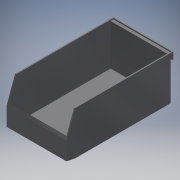
# Autodesk Inventor part: 22-124
Saved by Autodesk Inventor 2018 (Build 220105000, 105)
## iProperties
Created: 2004-11-24
Part Number: 22-124
Document SubType Name: Modeling
Designer: Autodesk, Inc.
Manufacturer: Standard
Standards Organization: Custom
Description: Parts Bin, Conductive, Small
Vendor: PARKER IPS
Catalog Web Link: http://www.parker.com/ead/cm1.asp?cmid=809
Mass: 114.974 g
Surface Area: 1166.8 cm^2
Volume: 114.974 cm^3
Density: 1 g/cm^3
Material: Generic
Appearance: Smooth - Medium Gray
CAGE: 1LJX3
Dept. ID: Product Design
Description #2: ---
Finish #1: ---
Finish #2: ---
Material ID: ---
Project Number: ---
Author: Autodesk, Inc.
Autodesk Inventor part; units mm, degrees
ref_plane "YZ Plane" through (0, 0, 0) normal (1, 0, 0) x (0, 1, 0)
ref_plane "XZ Plane" through (0, 0, 0) normal (0, 1, 0) x (-1, 0, 0)
ref_plane "XY Plane" through (0, 0, 0) normal (0, 0, 1) x (1, 0, 0)
sketch "Sketch2" plane through (0, 0, 0) normal (1, 0, 0) x (0, 1, 0)
  line L0 (-33.0843, 98.5) -> (-2.0843, 98.5)
  line L1 (-2.0843, 98.5) -> (40, 83.5)
  line L2 (40, 83.5) -> (40, -88.5)
  line L3 (40, -88.5) -> (28, -88.5)
  line L4 (28, -88.5) -> (28, -86.5)
  line L5 (28, -86.5) -> (36, -86.5)
  line L6 (36, -86.5) -> (36, -83.5)
  line L7 (36, -83.5) -> (-36, -83.5)
  line L8 (-36, -83.5) -> (-36, 83.5)
  line L9 (-36, 83.5) -> (-33.0843, 98.5)
  point P0 (0, 0)
  point P1 (0, -83.5)
  point P2 (-36, 0)
  dimension "d0" = 15
  dimension "d1" = 11
  dimension "d2" = 31
  dimension "d4" = 2
  dimension "d5" = 3
  dimension "d6" = 4
  dimension "d7" = 12
  dimension "Dim_D" = 187
  dimension "Dim_H" = 76
  dimension "d11" = 19.617
  dimension "d12" = 15
  constraints: 20 end point, 5 parallel, 2 midpoint, 2 perpendicular, 1 horizontal, 1 horizontal alignment, 1 vertical alignment
  measures "d0" vertical distance of L8.end L0.start
  measures "d1" angle of L8 L9
  measures "d2" distance of L0.start L0.end
  measures "d4" distance of L3.end L4.end
  measures "d5" distance between parallel lines of L7 L5
  measures "d6" distance between parallel lines of L2 L6
  measures "d7" distance of L2.end L3.end
  measures "Dim_D" distance between parallel lines of L3 L0
  measures "Dim_H" distance between parallel lines of L8 L2
  measures "d11" angle of L1 L0
  measures "d12" vertical distance of L0.end L1.end
extrude "Extrusion1" add sketch "Sketch2" along normal mid plane 105
shell "Shell1" thickness 2 removed faces 2 at (-17.5, 25.9719, 88.5) at (-17.5, 40, -31.1667)
body "Solid1"
